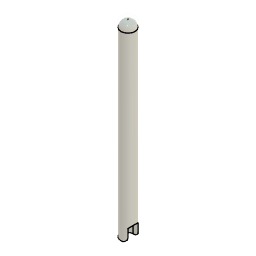
Antenna (Autodesk Fusion 360 archive; units mm, degrees)
design "Main Antenna Part"
Autodesk Fusion 360 part; units mm, degrees
note: some values were not read from the file. Set by a fixed rule: which face or edge a step refers to.
sketch "Sketch1" plane through (0, 0, 0) normal (0, 0, 1) x (1, 0, 0)
  circle A0 centre (0, 0) radius 6.75
  dimension "d1" = 13.5
  constraint coincident A0.centre origin
  measures "d1" diameter of A0
extrude "Extrude1" add sketch "Sketch1" along normal blind 177
sketch "Sketch2" plane through (0, 0, 177) normal (0, 0, 1) x (-1, 0, 0)
  circle A0 centre (0, 0) radius 6.75
fillet "Fillet1" radius 6.5 1 edges at (-6.2932, -2.4409, 177)
shell "Shell1" thickness 2 removed faces 1 at (-1.125, 1.9486, 0)
sketch "Sketch3" plane through (0, 0, 0) normal (1, 0, 0) x (0, 1, 0)
  line L0 (0, 0) -> (4.75, 0)
  line L1 (4.75, 0) -> (4.75, 11.5)
  line L2 (4.75, 11.5) -> (0, 11.5)
  line L3 (0, 11.5) -> (0, 0)
  line L4 (0, 14.5) -> (0, -2.5)
  line L5 (-4.75, 11.5) -> (0, 11.5)
  line L6 (-4.75, 0) -> (-4.75, 11.5)
  line L7 (0, 0) -> (-4.75, 0)
  dimension "d7" = 4.75
  dimension "d8" = 11.5
  constraint horizontal L0
  constraint vertical L1
  constraint horizontal L2
  constraint vertical L3
  constraint coincident L0.start L3.end
  constraint vertical L4
  constraint symmetric L0.start L4 L3.end
  constraint symmetric L0.end L4 L6.start
  constraint symmetric L1.end L4 L5.start
  constraint symmetric L2.end L4 L3.start
  measures "d7" distance of L0.start L0.end
  measures "d8" distance of L0.start L2.end
extrude "Extrude2" cut sketch "Sketch3" along normal blind 8.5
sketch "Sketch4" plane through (0, 4.75, 0) normal (0, -1, 0) x (1, 0, 0)
  line L0 (4.7958, 0) -> (4.7958, 11.5)
  line L1 (4.7958, 11.5) -> (0, 11.5)
  line L2 (0, 11.5) -> (0, 0)
  line L3 (0, 0) -> (4.7958, 0)
  line L4 (6.75, 170.5) -> (-6.75, 170.5)
  line L5 (4.7958, 0) -> (4.7958, 11.5)
  line L6 (6.75, 11.5) -> (4.7958, 11.5)
  line L7 (4.7958, 11.5) -> (4.7958, 0)
  line L8 (4.7958, 0) -> (-6.75, 0)
  line L9 (4.7958, 11.5) -> (7.626, 14.3302)
  line L10 (4.7958, 11.5) -> (8.7983, 11.5) construction
  line L11 (4.7958, 0) -> (4.7958, 4) construction
  line L12 (4.7958, 0) -> (0.7958, 0) construction
  arc A0 (0.7958, 0) -> (4.7958, 4) centre (0.9474, 3.8484) ccw
  line L13 (0.7958, 0) -> (3.6708, -2.6167)
  line L14 (3.6708, -2.6167) -> (7.087, -2.1687)
  line L15 (7.087, -2.1687) -> (8.8787, 5.4012)
  line L16 (8.8787, 5.4012) -> (10.2972, 10.4031)
  line L17 (10.2972, 10.4031) -> (8.8787, 14.6733)
  line L18 (8.8787, 14.6733) -> (7.626, 14.3302)
  line L19 (4.7958, 4) -> (4.7958, 11.5)
  dimension "d11" = 45
  dimension "d12" = 4
  dimension "d13" = 4
  constraint horizontal L10
  constraint coincident L0.end L1.start
  constraint coincident L0.start L3.end
  constraint perpendicular L8 L11
  constraint perpendicular L0 L12
  measures "d11" angle of L9 L10
  measures "d12" distance of L0.start L11.end
  measures "d13" distance of L0.start L12.end
extrude "Extrude3" cut sketch "Sketch4" along normal blind -5 and the other way blind -16 contours L0 L3 L5 L7 L8 L9 A0 L13 L14 L15 L16 L17 L18 L19 | L0 L3 L5 L7 L8 A0
equation "d7 = ( 9.5 / 2 ) * 1 mm"

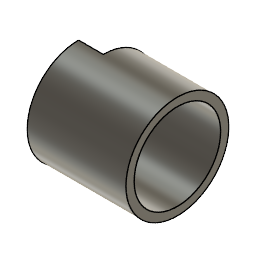
design "Antenna Connector part"
Autodesk Fusion 360 part; units mm, degrees
sketch "Sketch1" plane through (0, 0, 0) normal (1, 0, 0) x (0, 1, 0)
  circle A0 centre (0, 0) radius 6.25
  dimension "d1" = 12.5
  constraint coincident A0.centre origin
  measures "d1" diameter of A0
extrude "Extrude1" add sketch "Sketch1" along normal blind 12
shell "Shell1" thickness 1 removed faces 1 at (12, 0.0274, -1.4841)
extrude "Extrude2" cut 1 faces at (1, -0.9332, -1.2605) along direction (-1, 0, 0) blind 2.5
sketch "Sketch3" plane through (0, 0, 0) normal (-1, 0, 0) x (0, -1, 0)
  circle A0 centre (0, 0) radius 5.25
  circle A1 centre (0, 0) radius 6.25
  arc A2 (0, 6.25) -> (0, -6.25) centre (0, 0) ccw
  arc A3 (0, 5.25) -> (0, -5.25) centre (0, 0) ccw
  line L0 (0, 6.25) -> (0, 5.25)
  line L1 (0, -5.25) -> (0, -6.25)
  constraint coincident A1 A2.end
  constraint coincident A1 A2.start
  constraint coincident A0.centre A1.centre
  constraint coincident A0 A3.end
  constraint coincident A0 A3.start
  constraint vertical L0
  constraint parallel L0 L1
extrude "Extrude4" cut sketch "Sketch3" against normal blind 3 contours A0 A1 A2 A3 L0 L1
